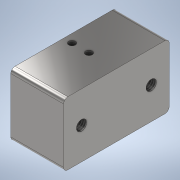
# Autodesk Inventor part: axle_tube_mount_8mm
Saved by Autodesk Inventor 2021.3 (Build 253353010, 353A)
## iProperties
Created: 2022-03-02
Part Number: axle_tube_mount_8mm
Material: Steel, Alloy
Document SubType Name: Modeling
Designer: au504769
Density: 7.73 g/cm^3
Appearance: Semi-Polished
Author: au504769
Autodesk Inventor part; units mm, degrees
ref_plane "YZ Plane" through (0, 0, 0) normal (1, 0, 0) x (0, 1, 0)
ref_plane "XZ Plane" through (0, 0, 0) normal (0, 1, 0) x (-1, 0, 0)
ref_plane "XY Plane" through (0, 0, 0) normal (0, 0, 1) x (1, 0, 0)
sketch "Sketch1" plane through (0, 0, 0) normal (1, 0, 0) x (0, 1, 0)
  line L0 (-15, 25) -> (15, 25)
  line L1 (15, 25) -> (15, -25)
  line L2 (15, -25) -> (-15, -25)
  line L3 (-15, -25) -> (-15, 25)
  line L4 (-15, 25) -> (15, -25) construction
  line L5 (15, 25) -> (-15, -25) construction
  point P0 (0, 0)
  dimension "d1" = 50
  dimension "d2" = 30
  constraints: 12 end point, 2 midpoint, 2 parallel, 1 horizontal, 1 perpendicular
  measures "d1" distance between parallel lines of L2 L0
  measures "d2" distance between parallel lines of L3 L1
extrude "Extrusion1" add sketch "Sketch1" along normal blind 25
hole "Hole1" at (0, 0, 0) direction (1, 0, 0) diameter 8 depth 20 tip angle 118
sketch "Sketch2" plane through (0, 15, 25) normal (0, 1, 0) x (1, 0, 0)
  line L0 (0, 25) -> (25, 25) construction
  line L1 (25, 50) -> (25, 0) construction
  line L2 (0, 50) -> (0, 0) construction
  point P0 (4, 25)
  point P1 (12, 25)
  dimension "d12" = 4
  dimension "d13" = 12
  constraints: 2 end point, 2 point on line, 1 midpoint
  measures "d12" distance from line of point (4, 25) L2
  measures "d13" distance from line of point (12, 25) L2
hole "Hole2" at (4, 15, 0) at (12, 15, 0) direction (0, -1, 0) diameter 3.242 end up to face face through (10, 0, 0) facing (1, 0, 0) round with radius 4 far side no thread size "M4x0.7" class "6H" standard "ISO Metric profile"
sketch "Sketch3" plane through (25, 0, 0) normal (1, 0, 0) x (0, 0, -1)
  line L0 (-16.5, 0) -> (0, 0) construction
  line L1 (0, 0) -> (16.5, 0) construction
  dimension "d21" = 33
  constraints: 4 end point, 2 collinear, 1 horizontal
  measures "d21" distance of L1.end L0.start
hole "Hole3" at (25, 0, 16.5) at (25, 0, -16.5) direction (-1, 0, 0) diameter 4.917 depth 17.1 tip angle 118 thread size "M6x1" class "6H" standard "ISO Metric profile"
fillet "Fillet1" radius 2 4 edges at (12.5, 15, -25) (12.5, -15, -25) (12.5, -15, 25) (12.5, 15, 25)
body "Solid1"
